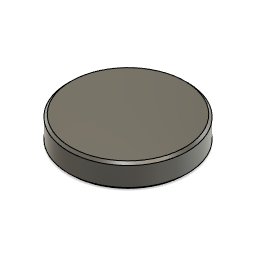
кубсат спарки (Autodesk Fusion 360 archive; units mm, degrees)
design "магнит 72 шт надо"
Autodesk Fusion 360 part; units mm, degrees
sketch "Sketch1" plane through (0, 0, 0) normal (0, 1, 0) x (1, 0, 0)
  circle A0 centre (0, 0) radius 2.5
  dimension "d1" = 5
  constraint coincident A0.centre origin
  measures "d1" diameter of A0
extrude "Extrude1" add sketch "Sketch1" along normal blind 1
chamfer "Chamfer1" distance 0.1 angle 45 2 edges at (-2.3308, 0, 0.904) (-2.3308, 1, 0.904)

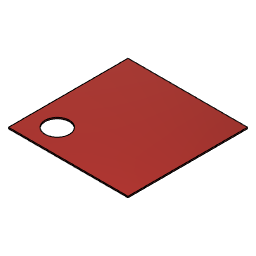
design "этаж"
Autodesk Fusion 360 part; units mm, degrees
sketch "Sketch1" plane through (0, 0, 0) normal (0, 1, 0) x (1, 0, 0)
  line L0 (0, 0) -> (98, 0)
  line L1 (98, 0) -> (98, 98)
  line L2 (98, 98) -> (0, 98)
  line L3 (0, 98) -> (0, 0)
  line L4 (0, 0) -> (15, 0)
  circle A0 centre (20, 20) radius 10
  dimension "d1" = 98
  dimension "d2" = 98
  constraint horizontal L0
  constraint vertical L1
  constraint horizontal L2
  constraint vertical L3
  constraint coincident L0.start L3.end
  constraint horizontal L4
  measures "d1" distance of L0.start L0.end
  measures "d2" distance of L0.start L2.end
extrude "Extrude1" add sketch "Sketch1" along normal blind 1
